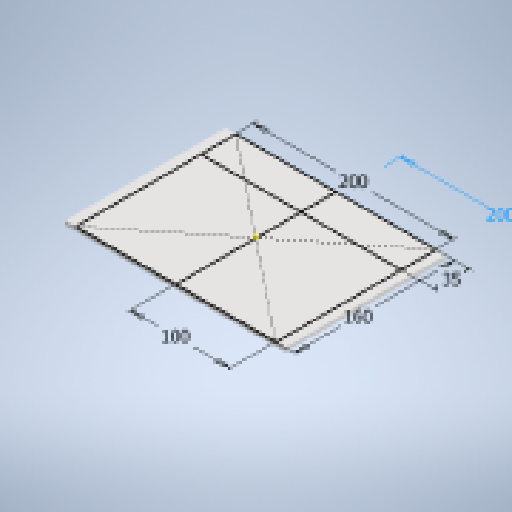
# Autodesk Inventor part: base
Saved by Autodesk Inventor 2023 (Build 270158000, 158)
## iProperties
Created: 2022-10-02
Part Number: base
Material: Generic
Document SubType Name: Modeling
Designer: carso
Density: 1 g/cm^3
Appearance: Default
Mass: 110 g
Surface Area: 577.6 cm^2
Volume: 110 cm^3
Author: carso
Autodesk Inventor part; units mm, degrees
ref_plane "YZ Plane" through (0, 0, 0) normal (1, 0, 0) x (0, 1, 0)
ref_plane "XZ Plane" through (0, 0, 0) normal (0, 1, 0) x (-1, 0, 0)
ref_plane "XY Plane" through (0, 0, 0) normal (0, 0, 1) x (1, 0, 0)
sketch "Sketch1" plane through (0, 0, 0) normal (0, 1, 0) x (-1, 0, 0)
  line L0 (-100, 80) -> (100, 80)
  line L1 (100, 80) -> (100, -80)
  line L2 (100, -80) -> (-100, -80)
  line L3 (-100, -80) -> (-100, 80)
  line L4 (-100, 80) -> (100, -80) construction
  line L5 (100, 80) -> (-100, -80) construction
  line L6 (-100, -45) -> (100, -45)
  line L7 (0, -80) -> (0, 80)
  point P0 (0, 0)
  dimension "d0" = 200
  dimension "d1" = 160
  dimension "d5" = 35
  dimension "d6" = 100
  constraints: 16 end point, 4 midpoint, 3 perpendicular, 2 parallel, 2 point on line, 1 horizontal
  measures "d0" distance of L1.end L2.end
  measures "d1" distance of L2.end L0.start
  measures "d5" distance between parallel lines of L2 L6
  measures "d6" distance between parallel lines of L3 L7
extrude "Extrusion1" add sketch "Sketch1" against normal blind 4
body "Solid1"
